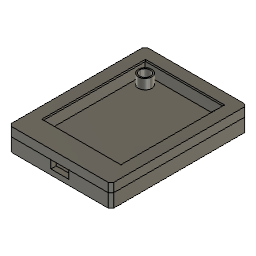
Bambu_watcher_enclosure (Autodesk Fusion 360 design; units mm, degrees)
part number: 2026-05-02-19-46-58-819
Autodesk Fusion 360 part; units mm, degrees
sketch "Sketch2" plane through (0, 0, 0) normal (0, 0, 1) x (1, 0, 0)
  line L0 (25.5, -35) -> (-25.5, -35)
  line L1 (-25.5, -35) -> (-25.5, 35)
  line L2 (-25.5, 35) -> (25.5, 35)
  line L3 (25.5, 35) -> (25.5, -35)
  line L4 (25.5, -35) -> (-25.5, 35) construction
  line L5 (-25.5, -35) -> (25.5, 35) construction
  circle A0 centre (-20.5, 30) radius 3
  line L6 (0, 1.75) -> (0, 22.5)
  circle A1 centre (20.5, 30) radius 3
  line L7 (1.75, 0) -> (22.5, 0)
  circle A2 centre (20.5, -30) radius 3
  circle A3 centre (-20.5, -30) radius 3
  line L8 (5, -35) -> (-5, -35)
  line L9 (-5, -35) -> (-5, -27.0284)
  line L10 (-5, -27.0284) -> (5, -27.0284)
  line L11 (5, -27.0284) -> (5, -35)
  circle A4 centre (-20.5, 30) radius 3.75
  circle A5 centre (20.5, 30) radius 3.75
  circle A6 centre (-20.5, -30) radius 3.75
  circle A7 centre (20.5, -30) radius 3.75
  line L12 (-28.5, -38) -> (-28.5, 38)
  line L13 (-28.5, 38) -> (28.5, 38)
  line L14 (28.5, 38) -> (28.5, -38)
  line L15 (28.5, -38) -> (-28.5, -38)
  line L16 (-5, -35) -> (-5, -38)
  line L17 (5, -35) -> (5, -38)
  line L18 (27, -36.5) -> (-27, -36.5)
  line L19 (-27, -36.5) -> (-27, 36.5)
  line L20 (-27, 36.5) -> (27, 36.5)
  line L21 (27, 36.5) -> (27, -36.5)
  line L22 (26.8, 36.3) -> (26.8, -36.3)
  line L23 (26.8, -36.3) -> (-26.8, -36.3)
  line L24 (-26.8, -36.3) -> (-26.8, 36.3)
  line L25 (-26.8, 36.3) -> (26.8, 36.3)
  line L26 (22, -26) -> (-22, -26)
  line L27 (-22, -26) -> (-22, 31.75)
  line L28 (-22, 31.75) -> (22, 31.75)
  line L29 (22, 31.75) -> (22, -26)
  point P0 (-22, 31.75)
  point P1 (22, -26)
  dimension "d1" = 51
  dimension "d2" = 70
  dimension "d3" = 6
  dimension "d4" = 5
  dimension "d5" = 5
  dimension "d6" = 20.5
  dimension "d7" = 10
  dimension "d8" = 0.75
  dimension "d9" = -3
  dimension "d18" = -1.5
  dimension "d22" = -1.3
  dimension "d33" = 3.25
  dimension "d34" = 3.5
  dimension "d35" = 3.5
  dimension "d36" = 9
  constraint horizontal L0
  constraint perpendicular L0 L1
  constraint parallel L0 L2
  constraint parallel L1 L3
  constraint coincident L4 origin
  constraint coincident L5 origin
  constraint symmetric A0 L6 A1
  constraint symmetric A0 L7 A3
  constraint symmetric A1 L7 A2
  constraint horizontal L8
  constraint vertical L9
  constraint horizontal L10
  constraint vertical L11
  constraint coincident L0 L8.start
  constraint symmetric L6 A4 A5
  constraint symmetric L7 A4 A6
  constraint symmetric L7 A5 A7
  constraint coincident L15 L16.end
  constraint perpendicular L15 L16
  constraint coincident L15 L17.end
  constraint perpendicular L15 L17
  constraint horizontal L26
  constraint vertical L27
  constraint horizontal L28
  constraint vertical L29
  constraint coincident P0 L27.end
  constraint coincident P1 L26.start
  measures "d1" distance of L1.end L2.end
  measures "d2" distance of L0.end L1.end
  measures "d3" diameter of A0
  measures "d4" distance of L2 A0.centre
  measures "d5" distance of L1 A0.centre
  measures "d6" distance of L0.start L8.start
  measures "d7" distance of L8.start L8.end
  measures "d33" distance of L2 P0
  measures "d34" distance of L1 P0
  measures "d35" distance of L3 P1
  measures "d36" distance of L0 P1
extrude "Extrude1" add sketch "Sketch2" along normal blind 2 contours L0 L1 L2 L3 L16 L17 L22 L23 L24 L25 | L0 L1 L2 L3 L9 L10 L11 | L0 L8 L16 L17 L23 | L0 L8 L9 L10 L11 | L16 L17 L18 L19 L20 L21 L22 L23 L24 L25 | L16 L17 L18 L23 | L12 L13 L14 L15 L16 L17 L18 L19 L20 L21 | L15 L16 L17 L18 | A0 L27 L28 | A0 A4 L27 L28 | A0 L27 L28 | A0 A4 L27 L28 | A4 A5 L26 L27 L28 L29 | A1 A5 L28 L29 | A1 A5 L28 L29 | A1 L28 L29 | A1 L28 L29 | A2 | A3 | A6 | A7 makes body 1
extrude "Extrude3" add sketch "Sketch2" along normal blind 5.5 from surface at 2 contours L0 L1 L2 L3 L16 L17 L22 L23 L24 L25 | L16 L17 L18 L19 L20 L21 L22 L23 L24 L25 | L12 L13 L14 L15 L16 L17 L18 L19 L20 L21 | A0 A4 L27 L28 | A0 A4 L27 L28 | A1 A5 L28 L29 | A1 A5 L28 L29 | A6 | A7 bodies 1
extrude "Extrude4" add sketch "Sketch2" along normal blind 4 from surface at 7.5 contours L0 L1 L2 L3 L16 L17 L22 L23 L24 L25 bodies 1
extrude "Extrude5" add sketch "Sketch2" along normal blind 1 from surface at 11.5 separate body contours L0 L1 L2 L3 L16 L17 L22 L23 L24 L25 | L0 L1 L2 L3 L9 L10 L11 | L0 L8 L16 L17 L23 | L0 L8 L9 L10 L11 | L16 L17 L18 L19 L20 L21 L22 L23 L24 L25 | L16 L17 L18 L23 | L12 L13 L14 L15 L16 L17 L18 L19 L20 L21 | L15 L16 L17 L18 | A0 L27 L28 | A0 A4 L27 L28 | A0 L27 L28 | A0 A4 L27 L28 | A4 A5 L26 L27 L28 L29 | A1 A5 L28 L29 | A1 A5 L28 L29 | A1 L28 L29 | A1 L28 L29 | A2 | A3 | A6 | A7 makes body 2
extrude "Extrude6" add sketch "Sketch2" against normal blind 4 from surface at 11.5 contours L12 L13 L14 L15 L16 L17 L18 L19 L20 L21 | L15 L16 L17 L18 bodies 2
chamfer "Chamfer1" distance 1.5 angle 45 8 edges at (28.5, -38, 3.75) (-28.5, -38, 3.75) (-28.5, 38, 3.75) (28.5, 38, 3.75) (28.5, -38, 10) (-28.5, -38, 10) (-28.5, 38, 10) (28.5, 38, 10) on bodies 1 2
extrude "Extrude9" cut sketch "Sketch2" against normal up to surface (1 mm away) from surface at 12.5 contours A0 L27 L28 | A0 A4 L27 L28 | A4 A5 L26 L27 L28 L29 | A1 A5 L28 L29 | A1 L28 L29 picked at (-19.6435, 29.1213) picked at (-19.7195, 26.5946) picked at (21.7005, 26.72) picked at (19.7271, 29.0473) bodies 2
extrude "Extrude10" add sketch "Sketch2" along normal blind 1 from surface at 2 contours L0 L8 L16 L17 L23 | L16 L17 L18 L23 | L15 L16 L17 L18 bodies 1
sketch "Sketch3" plane through (26.8, 0, 0) normal (1, 0, 0) x (0, 1, 0)
  line L0 (-36.3, 7.5) -> (36.3, 7.5)
  line L1 (36.3, 7.5) -> (36.3, 11.5)
  line L2 (36.3, 11.5) -> (-36.3, 11.5)
  line L3 (-36.3, 11.5) -> (-36.3, 7.5)
  line L4 (0, 1.75) -> (0, 22.5)
  line L5 (21.15, 8.5) -> (21.15, 10.5)
  line L6 (15.15, 8.5) -> (21.15, 8.5)
  line L7 (21.15, 10.5) -> (15.15, 10.5)
  line L8 (15.15, 10.5) -> (15.15, 8.5)
  line L9 (-36.3, 9.5) -> (0, 9.5)
  line L10 (1.75, 0) -> (22.5, 0)
  line L11 (-30.25, 11.5) -> (-30.25, 7.5) construction
  line L12 (-6.05, 11.5) -> (-6.05, 7.5) construction
  line L13 (-18.15, 11.5) -> (-18.15, 7.5) construction
  line L14 (-27.25, 10.5) -> (-33.25, 10.5)
  line L15 (-33.25, 10.5) -> (-33.25, 8.5)
  line L16 (-33.25, 8.5) -> (-27.25, 8.5)
  line L17 (-27.25, 8.5) -> (-27.25, 10.5)
  line L18 (-27.25, 10.5) -> (-33.25, 8.5) construction
  line L19 (-33.25, 10.5) -> (-27.25, 8.5) construction
  line L20 (-15.15, 8.5) -> (-21.15, 8.5)
  line L21 (-21.15, 8.5) -> (-21.15, 10.5)
  line L22 (-21.15, 10.5) -> (-15.15, 10.5)
  line L23 (-15.15, 10.5) -> (-15.15, 8.5)
  line L24 (-15.15, 8.5) -> (-21.15, 10.5) construction
  line L25 (-21.15, 8.5) -> (-15.15, 10.5) construction
  line L26 (-3.05, 8.5) -> (-9.05, 8.5)
  line L27 (-9.05, 8.5) -> (-9.05, 10.5)
  line L28 (-9.05, 10.5) -> (-3.05, 10.5)
  line L29 (-3.05, 10.5) -> (-3.05, 8.5)
  line L30 (-3.05, 8.5) -> (-9.05, 10.5) construction
  line L31 (-9.05, 8.5) -> (-3.05, 10.5) construction
  line L32 (9.05, 10.5) -> (3.05, 10.5)
  line L33 (9.05, 8.5) -> (3.05, 10.5) construction
  line L34 (6.05, 11.5) -> (6.05, 7.5) construction
  line L35 (3.05, 8.5) -> (9.05, 8.5)
  line L36 (36.3, 9.5) -> (0, 9.5)
  line L37 (3.05, 10.5) -> (3.05, 8.5)
  line L38 (9.05, 8.5) -> (9.05, 10.5)
  line L39 (15.15, 10.5) -> (15.15, 8.5)
  line L40 (21.15, 8.5) -> (21.15, 10.5)
  line L41 (21.15, 10.5) -> (15.15, 10.5)
  line L42 (15.15, 8.5) -> (21.15, 8.5)
  line L43 (33.25, 8.5) -> (27.25, 8.5)
  line L44 (27.25, 8.5) -> (27.25, 10.5)
  line L45 (27.25, 10.5) -> (33.25, 10.5)
  line L46 (33.25, 10.5) -> (33.25, 8.5)
  point P0 (-36.3, 9.5)
  point P1 (-30.25, 9.5)
  point P2 (-24.2, 9.5)
  point P3 (-18.15, 9.5)
  point P4 (-12.1, 9.5)
  point P5 (-6.05, 9.5)
  point P6 (0, 9.5)
  point P7 (-30.25, 9.5)
  point P8 (-18.15, 9.5)
  point P9 (-6.05, 9.5)
  dimension "d74" = 36.3
  dimension "d75" = 0
  dimension "d76" = 6
  dimension "d77" = 2
  dimension "d78" = 6
  dimension "d79" = 2
  dimension "d80" = 6
  dimension "d81" = 2
  constraint midpoint L3 P0
  constraint coincident L4 P6
  constraint perpendicular L4 L9
  constraint coincident P0 L9.start
  constraint coincident L2 L11.start
  constraint coincident L0 L11.end
  constraint perpendicular L0 L11
  constraint coincident L2 L12.start
  constraint coincident L0 L12.end
  constraint perpendicular L0 L12
  constraint coincident L2 L13.start
  constraint coincident L0 L13.end
  constraint perpendicular L0 L13
  constraint horizontal L14
  constraint perpendicular L14 L15
  constraint parallel L14 L16
  constraint parallel L15 L17
  constraint coincident L18 P7
  constraint coincident L19 P7
  constraint coincident P7 P1
  constraint horizontal L20
  constraint perpendicular L20 L21
  constraint parallel L20 L22
  constraint parallel L21 L23
  constraint coincident L24 P8
  constraint coincident L25 P8
  constraint coincident P8 P3
  constraint horizontal L26
  constraint perpendicular L26 L27
  constraint parallel L26 L28
  constraint parallel L27 L29
  constraint coincident L30 P9
  constraint coincident L31 P9
  constraint coincident P9 P5
  constraint symmetric L4 P0 L36.start
  constraint symmetric L4 P6 L9.end
  constraint symmetric L4 L12.start L34.start
  constraint symmetric L4 L12.end L34.end
  constraint symmetric L4 L14.start L44.end
  constraint symmetric L4 L14.end L45.end
  constraint symmetric L4 L15.end L43.start
  constraint symmetric L4 L16.end L43.end
  constraint symmetric L4 L20.start L6.start
  constraint symmetric L4 L20.end L5.start
  constraint symmetric L4 L21.end L5.end
  constraint symmetric L4 L22.end L7.end
  constraint symmetric L4 L26.start L35.start
  constraint symmetric L4 L26.end L33.start
  constraint symmetric L4 L27.end L32.start
  constraint symmetric L4 L28.end L32.end
  measures "d76" distance of L15.end L16.end
  measures "d77" distance of L14.end L15.end
  measures "d78" distance of L21.end L22.end
  measures "d79" distance of L20.end L21.end
  measures "d80" distance of L27.end L28.end
  measures "d81" distance of L26.end L27.end
extrude "Extrude11" add sketch "Sketch3" along normal blind 1 draft -48 contours L9 L14 L15 L17 | L9 L15 L16 L17 | L9 L26 L27 L29 | L9 L27 L28 L29 | L32 L36 L37 L38 | L35 L36 L37 L38 | L36 L43 L44 L46 | L36 L44 L45 L46 | L9 L21 L22 L23 | L9 L20 L21 L23 | L5 L6 L8 L36 L39 L40 L42 | L5 L7 L8 L36 L39 L40 L41 bodies 1
mirror "Mirror1" about plane through (0, 0, 0) normal (1, 0, 0) of "Extrude11"
sketch "Sketch5" plane through (27, 0, 0) normal (-1, 0, 0) x (0, -1, 0)
  line L0 (36.5, 11.5) -> (-36.5, 11.5)
  line L1 (-36.5, 11.5) -> (-36.5, 7.5)
  line L2 (-36.5, 7.5) -> (36.5, 7.5)
  line L3 (36.5, 7.5) -> (36.5, 11.5)
  line L4 (-21.15, 8.5) -> (-21.15, 10.5)
  line L5 (-15.15, 10.5) -> (-15.15, 8.5)
  line L6 (27.25, 10.5) -> (33.25, 10.5)
  line L7 (33.25, 8.5) -> (27.25, 8.5)
  line L8 (27.25, 8.5) -> (27.25, 10.5)
  line L9 (33.25, 10.5) -> (33.25, 8.5)
  line L10 (3.05, 8.5) -> (9.05, 8.5)
  line L11 (9.05, 8.5) -> (9.05, 10.5)
  line L12 (9.05, 10.5) -> (3.05, 10.5)
  line L13 (3.05, 10.5) -> (3.05, 8.5)
  line L14 (21.15, 10.5) -> (15.15, 10.5)
  line L15 (21.15, 8.5) -> (21.15, 10.5)
  line L16 (15.15, 8.5) -> (21.15, 8.5)
  line L17 (15.15, 10.5) -> (15.15, 8.5)
  line L18 (-9.05, 10.5) -> (-3.05, 10.5)
  line L19 (-9.05, 8.5) -> (-9.05, 10.5)
  line L20 (-3.05, 8.5) -> (-9.05, 8.5)
  line L21 (-3.05, 10.5) -> (-3.05, 8.5)
  line L22 (-21.15, 10.5) -> (-15.15, 10.5)
  line L23 (-21.15, 8.5) -> (-21.15, 10.5)
  line L24 (-15.15, 8.5) -> (-21.15, 8.5)
  line L25 (-36.3, 9.5) -> (0, 9.5)
  line L26 (-27.25, 10.5) -> (-33.25, 10.5)
  line L27 (-33.25, 8.5) -> (-27.25, 8.5)
  line L28 (-27.25, 8.5) -> (-27.25, 10.5)
  line L29 (-33.25, 10.5) -> (-33.25, 8.5)
  line L30 (-15.15, 10.5) -> (-15.15, 8.5)
extrude "Extrude13" cut sketch "Sketch5" against normal blind 1 draft -48 contours L4 L5 L23 L24 L25 L30 | L4 L5 L22 L23 L25 L30 | L6 L7 L8 L9 | L10 L11 L12 L13 | L14 L15 L16 L17 | L18 L19 L21 L25 | L19 L20 L21 L25 | L25 L26 L28 L29 | L25 L27 L28 L29 bodies 2
mirror "Mirror2" about plane through (0, 0, 0) normal (1, 0, 0) of "Extrude13"
sketch "Sketch7" plane through (0, -36.3, 0) normal (0, -1, 0) x (1, 0, 0)
  line L0 (-26.8, 7.5) -> (-5, 7.5)
  line L1 (-5, 7.5) -> (-5, 11.5)
  line L2 (-5, 11.5) -> (-26.8, 11.5)
  line L3 (-26.8, 11.5) -> (-26.8, 7.5)
  line L4 (-26.8, 11.5) -> (-5, 7.5)
  line L5 (-26.8, 7.5) -> (-5, 11.5)
  line L6 (-12.9, 8.5) -> (-18.9, 8.5)
  line L7 (-18.9, 8.5) -> (-18.9, 10.5)
  line L8 (-18.9, 10.5) -> (-12.9, 10.5)
  line L9 (-12.9, 10.5) -> (-12.9, 8.5)
  line L10 (-12.9, 8.5) -> (-18.9, 10.5) construction
  line L11 (-18.9, 8.5) -> (-12.9, 10.5) construction
  line L12 (0, 1.75) -> (0, 22.5)
  line L13 (12.9, 8.5) -> (18.9, 8.5)
  line L14 (18.9, 10.5) -> (12.9, 10.5)
  line L15 (18.9, 8.5) -> (18.9, 10.5)
  line L16 (12.9, 10.5) -> (12.9, 8.5)
  point P0 (-15.9, 9.5)
  dimension "d62" = 6
  dimension "d63" = 2
  constraint coincident L2.end L3.start
  constraint coincident L0.end L1.start
  constraint coincident L0.start L3.end
  constraint coincident L1.end L2.start
  constraint horizontal L6
  constraint perpendicular L6 L7
  constraint parallel L6 L8
  constraint parallel L7 L9
  constraint coincident L10 P0
  constraint coincident L11 P0
  constraint midpoint L4 P0
  constraint symmetric L6.start L12 L13.start
  constraint symmetric L6.end L12 L13.end
  constraint symmetric L7.end L12 L14.start
  constraint symmetric L8.end L12 L14.end
  measures "d62" distance of L7.end L8.end
  measures "d63" distance of L6.end L7.end
extrude "Extrude14" add sketch "Sketch7" along normal blind 1 draft -48 contours L4 L5 L7 | L4 L5 L6 L7 L9 | L4 L5 L9 | L4 L5 L7 L8 L9 | L13 L14 L15 L16 bodies 1
mirror "Mirror3" about plane through (0, 0, 0) normal (0, 1, 0) of "Extrude14"
sketch "Sketch8" plane through (0, -36.5, 0) normal (0, 1, 0) x (-1, 0, 0)
  line L0 (27, 11.5) -> (-27, 11.5)
  line L1 (-27, 11.5) -> (-27, 7.5)
  line L2 (-27, 7.5) -> (27, 7.5)
  line L3 (27, 7.5) -> (27, 11.5)
  line L4 (-18.9, 10.5) -> (-12.9, 10.5)
  line L5 (-18.9, 8.5) -> (-18.9, 10.5)
  line L6 (-12.9, 8.5) -> (-18.9, 8.5)
  line L7 (-12.9, 10.5) -> (-12.9, 8.5)
  line L8 (12.9, 10.5) -> (12.9, 8.5)
  line L9 (18.9, 10.5) -> (12.9, 10.5)
  line L10 (18.9, 8.5) -> (18.9, 10.5)
  line L11 (12.9, 8.5) -> (18.9, 8.5)
extrude "Extrude15" cut sketch "Sketch8" against normal blind 1 draft -48 contours L4 L5 L6 L7 | L8 L9 L10 L11 bodies 2
mirror "Mirror4" about plane through (0, 0, 0) normal (0, 1, 0) of "Extrude15"
equation "d33 = 1.5 mm + 1.75 mm"
equation "d34 = 2.75 mm + 0.75 mm"
equation "d35 = 2.75 mm + 0.75 mm"
named bodies: "Case", "Lid"
